z_motor_holder_left (Autodesk Fusion 360 design; units mm, degrees)
Autodesk Fusion 360 part; units mm, degrees
note: some values were not read from the file. Chosen so that the rebuilt part matches the saved one: which face or edge a step refers to; which pieces of a blend or face edit are solid.
sketch "Sketch1" plane through (0, 0, 0) normal (0, 0, 1) x (1, 0, 0)
  line L0 (0, 0) -> (53.3, 0)
  line L1 (83.3, 50.3) -> (0, 50.3)
  line L2 (0, 50.3) -> (0, 0)
  line L3 (53.3, 20.3) -> (83.3, 20.3)
  line L4 (83.3, 20.3) -> (83.3, 50.3)
  line L5 (53.3, 20.3) -> (53.3, 0)
  circle A0 centre (68.3, 35.3) radius 2.6
  circle A1 centre (8.65, 36.65) radius 1.6
  circle A2 centre (39.65, 36.65) radius 1.6
  circle A3 centre (39.65, 5.65) radius 1.6
  circle A4 centre (8.65, 5.65) radius 1.6
  circle A5 centre (24.15, 21.15) radius 11.5
  line L6 (8.65, 36.65) -> (39.65, 5.65) construction
  circle A6 centre (7.15, 21.15) radius 4
  dimension "d2" = 50.3
  dimension "d3" = 53.3
  dimension "d4" = 5.2
  dimension "d5" = 15
  dimension "d6" = 30
  dimension "d7" = 15
  dimension "d8" = 15
  dimension "d9" = 3.2
  dimension "d10" = 31
  dimension "d11" = 31
  dimension "d12" = 5.65
  dimension "d13" = 8.65
  dimension "d31" = 23
  dimension "d32" = 8
  dimension "d33" = 17
  constraint horizontal L0
  constraint horizontal L1
  constraint vertical L2
  constraint coincident L0.start L2.end
  constraint horizontal L3
  constraint vertical L4
  constraint perpendicular L0 L5
  constraint equal A1 A4
  constraint equal A1 A2
  constraint equal A2 A3
  constraint horizontal A1.centre A2.centre
  constraint vertical A2.centre A3.centre
  constraint vertical A1.centre A4.centre
  constraint horizontal A3.centre A4.centre
  constraint coincident A1.centre L6.start
  constraint coincident A3.centre L6.end
  constraint midpoint A5.centre L6
  constraint horizontal A5.centre A6.centre
  measures "d2" distance of L0.start L1.end
  measures "d3" distance of L0.start L0.end
  measures "d4" diameter of A0
  measures "d5" distance of L5 A0.centre
  measures "d6" distance of L1.start L3.end
  measures "d7" distance of L1 A0.centre
  measures "d8" distance of L4 A0.centre
  measures "d9" diameter of A1
  measures "d10" distance of A1.centre A2.centre
  measures "d11" vertical distance of A1.centre A4.centre
  measures "d12" distance of L0 A4.centre
  measures "d13" distance of L2 A4.centre
  measures "d31" diameter of A5
  measures "d32" diameter of A6
  measures "d33" horizontal distance of A5.centre A6.centre
extrude "Extrude1" add sketch "Sketch1" against normal blind 4
sketch "Sketch2" plane through (0, 0, -4) normal (0, 0, -1) x (1, 0, 0)
  circle A0 centre (8.65, -5.65) radius 1.6
  circle A1 centre (39.65, -36.65) radius 1.6
  circle A2 centre (39.65, -5.65) radius 1.6
  circle A3 centre (8.65, -36.65) radius 1.6
  circle A4 centre (68.3, -35.3) radius 2.6
  line L0 (83.3, -50.3) -> (83.3, -20.3)
  line L1 (83.3, -20.3) -> (53.3, -20.3)
  line L2 (53.3, -20.3) -> (53.3, 0)
  line L3 (53.3, 0) -> (0, 0)
  line L4 (0, 0) -> (0, -50.3)
  line L5 (0, -50.3) -> (83.3, -50.3)
  line L6 (53.3, -20.3) -> (53.3, -50.3)
  circle A5 centre (7.15, -21.15) radius 4
  circle A6 centre (24.15, -21.15) radius 11.5
  constraint coincident L1.end L2.start
  constraint coincident L5 L6.end
  constraint perpendicular L5 L6
extrude "Extrude2" add sketch "Sketch2" along normal blind 15 contours L0 L1 L5 L6
sketch "Sketch3" plane through (0, 0, -4) normal (0, 0, -1) x (1, 0, 0)
  line L0 (53.3, -50.3) -> (53.3, -20.3)
  line L1 (53.3, -20.3) -> (53.3, 0)
  line L2 (53.3, 0) -> (0, 0)
  line L3 (0, 0) -> (0, -50.3)
  line L4 (0, -50.3) -> (53.3, -50.3)
  circle A0 centre (8.65, -36.65) radius 1.6
  circle A1 centre (39.65, -5.65) radius 1.6
  circle A2 centre (39.65, -36.65) radius 1.6
  circle A3 centre (8.65, -5.65) radius 1.6
  line L5 (0, -42.4) -> (45.4, -42.4)
  line L6 (45.4, -42.4) -> (45.4, 0)
  circle A4 centre (24.15, -21.15) radius 11.5
  circle A5 centre (7.15, -21.15) radius 4
  dimension "d18" = 7.9
  dimension "d19" = 7.9
  constraint coincident L3 L5.start
  constraint perpendicular L3 L5
  constraint coincident L2 L6.end
  constraint perpendicular L2 L6
  measures "d18" distance of L1 L6
  measures "d19" distance of L4 L5
extrude "Extrude3" add sketch "Sketch3" along normal blind 40 contours L0 L1 L2 L3 L4 L5 L6
sketch "Sketch4" plane through (53.3, 0, 0) normal (1, 0, 0) x (0, 1, 0)
  line L0 (20.3, 0) -> (0, 0)
  line L1 (0, 0) -> (0, -44)
  line L2 (0, -44) -> (50.3, -44)
  line L3 (50.3, -44) -> (50.3, -19)
  line L4 (50.3, -19) -> (20.3, -19)
  line L5 (20.3, -19) -> (20.3, 0)
  circle A0 centre (21.15, -34) radius 1.6
  circle A1 centre (21.15, -34) radius 3.25
  dimension "d22" = 3.2
  dimension "d23" = 6.5
  dimension "d24" = 15
  dimension "d25" = 21.15
  constraint concentric A0 A1
  measures "d22" diameter of A0
  measures "d23" diameter of A1
  measures "d24" distance of L4 A0.centre
  measures "d25" distance of L1 A0.centre
extrude "Extrude4" cut sketch "Sketch4" against normal through all contours A0
extrude "Extrude5" cut sketch "Sketch4" along normal blind 3.2 from surface at -7.9 contours A1
sketch "Sketch5" plane through (0, 42.4, 0) normal (0, -1, 0) x (1, 0, 0)
  line L0 (45.4, -4) -> (0, -4)
  line L1 (0, -4) -> (0, -44)
  line L2 (0, -44) -> (45.4, -44)
  line L3 (45.4, -44) -> (45.4, -4)
  line L4 (0, -4) -> (45.4, -44)
  constraint coincident L0.end L1.start
  constraint coincident L2.end L3.start
extrude "Extrude6" cut sketch "Sketch5" against normal through all contours L1 L2 L4
sketch "Sketch6" plane through (0, 0, 0) normal (0, 0, 1) x (-1, 0, 0)
  circle A0 centre (-39.65, -36.65) radius 1.6
  circle A1 centre (-68.3, -35.3) radius 2.6
  circle A2 centre (-39.65, -5.65) radius 1.6
  circle A3 centre (-8.65, -5.65) radius 1.6
  circle A4 centre (-8.65, -36.65) radius 1.6
  circle A5 centre (-24.15, -21.15) radius 11.5
  circle A6 centre (-7.15, -21.15) radius 4
  line L0 (-83.3, -20.3) -> (-83.3, -50.3)
  line L1 (-83.3, -50.3) -> (0, -50.3)
  line L2 (0, -50.3) -> (0, 0)
  line L3 (0, 0) -> (-53.3, 0)
  line L4 (-53.3, 0) -> (-53.3, -20.3)
  line L5 (-53.3, -20.3) -> (-83.3, -20.3)
  circle A7 centre (-7.15, -21.15) radius 6.5
  circle A8 centre (-68.3, -35.3) radius 7
  dimension "d34" = 13
  dimension "d35" = 14
  constraint concentric A6 A7
  constraint concentric A1 A8
  measures "d34" diameter of A7
  measures "d35" diameter of A8
extrude "Extrude7" add sketch "Sketch6" along normal blind 3 contours A5 A7 picked at (-11.9914, -24.066)
chamfer "Chamfer1" distance 2 angle 45 2 edges at (5.6998, 14.8138, 0) (5.6998, 27.4862, 0)
fillet "Fillet1" radius 3 6 edges at (0, 50.3, -2) (0, 0, -2) (53.3, 0, -22) (53.3, 20.3, -9.5) (83.3, 20.3, -9.5) (83.3, 50.3, -9.5)
sketch "Sketch7" plane through (0, 0, 0) normal (0, 0, 1) x (-1, 0, 0)
  circle A0 centre (-8.65, -36.65) radius 1.6
  circle A1 centre (-8.65, -5.65) radius 1.6
  circle A2 centre (-39.65, -5.65) radius 1.6
  circle A3 centre (-39.65, -36.65) radius 1.6
  arc A4 (-83.3, -47.3) -> (-80.3, -50.3) centre (-80.3, -47.3) ccw
  line L0 (-80.3, -50.3) -> (-3, -50.3)
  arc A5 (-3, -50.3) -> (0, -47.3) centre (-3, -47.3) ccw
  line L1 (0, -47.3) -> (0, -25.7465)
  arc A6 (-13.8853, -26.3352) -> (0, -25.7465) centre (-7.15, -21.15) ccw
  arc A7 (-13.8853, -15.9648) -> (-13.8853, -26.3352) centre (-24.15, -21.15) ccw
  arc A8 (0, -16.5535) -> (-13.8853, -15.9648) centre (-7.15, -21.15) ccw
  line L2 (0, -16.5535) -> (0, -3)
  arc A9 (0, -3) -> (-3, 0) centre (-3, -3) ccw
  line L3 (-3, 0) -> (-50.3, 0)
  arc A10 (-50.3, 0) -> (-53.3, -3) centre (-50.3, -3) ccw
  line L4 (-53.3, -3) -> (-53.3, -17.3)
  arc A11 (-56.3, -20.3) -> (-53.3, -17.3) centre (-56.3, -17.3) ccw
  line L5 (-56.3, -20.3) -> (-80.3, -20.3)
  arc A12 (-80.3, -20.3) -> (-83.3, -23.3) centre (-80.3, -23.3) ccw
  line L6 (-83.3, -23.3) -> (-83.3, -47.3)
  circle A13 centre (-68.3, -35.3) radius 2.6
  line L7 (-53.3, -17.3) -> (-53.3, -50.3)
  constraint coincident L4.end A11.end
  constraint coincident L0 L7.end
  constraint perpendicular L0 L7
extrude "Extrude9" cut sketch "Sketch7" against normal blind 10 contours A0 | A1 | A2 | A3 | A4 L0 A11 L5 A12 L6 L7
fillet "Fillet2" radius 7 1 edges at (53.3, 33.8, -10)
sketch "Sketch8" plane through (0, 42.4, 0) normal (0, -1, 0) x (1, 0, 0)
  line L0 (0, -4) -> (45.4, -44)
  line L1 (45.4, -44) -> (45.4, -4)
  circle A0 centre (38.2, -19) radius 3
  circle A1 centre (38.2, -19) radius 1.6
  line L2 (45.4, -4) -> (0, -4)
  line L3 (53.3, -44) -> (53.3, 0)
  dimension "d47" = 3.2
  dimension "d48" = 6
  dimension "d54" = 15.1
  dimension "d55" = 15
  constraint concentric A0 A1
  measures "d47" diameter of A1
  measures "d48" diameter of A0
  measures "d54" distance of A0.centre L3
  measures "d55" distance of A0.centre L2
extrude "Extrude10" cut sketch "Sketch8" against normal through all contours A1
extrude "Extrude11" cut sketch "Sketch8" against normal blind 3.2 contours A0
equation "d2 = 42.3 mm + 8 mm"
equation "d3 = 42.3 mm + 8 mm + 3 mm"
equation "d7 = d5"
equation "d8 = d5"
equation "d11 = d10"
equation "d12 = ( ( 42.3 - 31 ) / 2 ) * 1 mm"
equation "d13 = d12 + 3 mm"
equation "d18 = d19"
equation "d25 = ( 42.3 / 2 ) * 1 mm"
